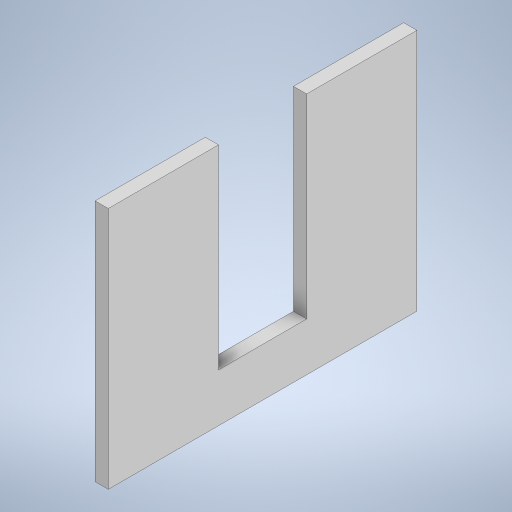
# Autodesk Inventor part: xd
Saved by Autodesk Inventor 2023 (Build 270158000, 158)
## iProperties
Created: 2022-11-03
Part Number: xd
Material: Generic
Document SubType Name: Modeling
Designer: diego
Density: 1 g/cm^3
Appearance: Default
Author: diego
Autodesk Inventor part; units mm, degrees
ref_plane "YZ Plane" through (0, 0, 0) normal (1, 0, 0) x (0, 1, 0)
ref_plane "XZ Plane" through (0, 0, 0) normal (0, 1, 0) x (-1, 0, 0)
ref_plane "XY Plane" through (0, 0, 0) normal (0, 0, 1) x (1, 0, 0)
sketch "Sketch1" plane through (0, 0, 0) normal (1, 0, 0) x (0, 1, 0)
  line L0 (0, 0) -> (0, -70)
  line L1 (0, 0) -> (55.175, 0)
  line L2 (55.175, 0) -> (55.175, -25)
  line L3 (55.175, -25) -> (10.975, -25)
  line L4 (10.975, -25) -> (10.975, -45)
  line L5 (10.975, -45) -> (55.175, -45)
  line L6 (55.175, -45) -> (55.175, -70)
  line L7 (55.175, -70) -> (0, -70)
  dimension "d0" = 70
  dimension "d4" = 55.175
  dimension "d5" = 25
  dimension "d6" = 44.2
  dimension "d7" = 20
  dimension "d8" = 25
  constraints: 16 end point, 3 perpendicular, 3 vertical, 2 horizontal
  measures "d0" distance of L0.start L0.end
  measures "d4" distance of L0.start L1.end
  measures "d5" distance of L1.end L2.end
  measures "d6" distance of L2.end L3.end
  measures "d7" distance of L3.end L4.end
  measures "d8" distance of L5.end L6.end
extrude "Extrusion1" add sketch "Sketch1" along normal blind 3
body "Solid1"
